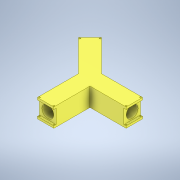
# Autodesk Inventor part: testPrintBracket
Saved by Autodesk Inventor 2022 (Build 260153000, 153)
## iProperties
Created: 2022-02-05
Part Number: testPrintBracket
Material: Generic
Document SubType Name: Modeling
Designer: ultra
Density: 1 g/cm^3
Appearance: Smooth - Yellow
Author: ultra
Autodesk Inventor part; units mm, degrees
ref_plane "YZ Plane" through (0, 0, 0) normal (1, 0, 0) x (0, 1, 0)
ref_plane "XZ Plane" through (0, 0, 0) normal (0, 1, 0) x (-1, 0, 0)
ref_plane "XY Plane" through (0, 0, 0) normal (0, 0, 1) x (1, 0, 0)
sketch "Sketch2" plane through (0, 0, 0) normal (1, 0, 0) x (0, 1, 0)
  circle A0 centre (0, 0) radius 13.2937
  line L0 (-16, -18.5) -> (16, -18.5)
  line L1 (16, -18.5) -> (16, 18.5)
  line L2 (16, 18.5) -> (-16, 18.5)
  line L3 (-16, 18.5) -> (-16, -18.5)
  line L4 (-16, -18.5) -> (16, 18.5) construction
  line L5 (16, -18.5) -> (-16, 18.5) construction
  dimension "d9" = 26.5875
  dimension "d10" = 32
  dimension "d11" = 37
  constraints: 12 end point, 2 midpoint, 2 parallel, 1 centre point, 1 coincident, 1 horizontal, 1 perpendicular
  measures "d9" diameter of A0
  measures "d10" distance of L2.end L1.end
  measures "d11" distance of L1.end L0.end
extrude "Extrusion2" add sketch "Sketch2" along normal blind 76.2
sketch "Sketch3" plane through (0, -16, -18.5) normal (0, 0, -1) x (-1, 0, 0)
  line L0 (0, 0) -> (0, 32) projected
  circle A0 centre (18.5, 16) radius 13.2937
  line L1 (0, 32) -> (0, 0)
  line L2 (0, 0) -> (37, 0)
  line L3 (37, 0) -> (37, 32)
  line L4 (37, 32) -> (0, 32)
  line L5 (0, 32) -> (37, 0) construction
  line L6 (0, 0) -> (37, 32) construction
  point P0 (0, 16)
  dimension "d14" = 26.5875
  dimension "d15" = 32
  dimension "d16" = 37
  constraints: 12 end point, 2 midpoint, 2 parallel, 1 centre point, 1 coincident, 1 perpendicular
  measures "d14" diameter of A0
  measures "d15" distance of L3.end L2.end
  measures "d16" distance of L2.end L1.end
extrude "Extrusion3" add sketch "Sketch3" against normal blind 113.2
sketch "Sketch4" plane through (76.2, -16, -18.5) normal (0, 0, -1) x (-1, 0, 0)
  circle A0 centre (94.7, 16) radius 13.2937 projected
  point P0 (76.2, 16)
extrude "Extrusion4" add sketch "Sketch4" against normal blind 37
sketch "Sketch5" plane through (76.2, 16, 18.5) normal (0, 1, 0) x (1, 0, 0)
  line L0 (-113.2, 37) -> (0, 37) projected
  line L1 (-113.2, 37) -> (-113.2, -76.2) projected
  line L2 (-113.2, 37) -> (-100.1185, 50.0815)
  line L3 (-113.2, 37) -> (-94.7, 37) construction
  line L4 (-113.2, 37) -> (-126.2815, 23.9185)
  line L5 (-113.2, 37) -> (-94.7, 37) construction
  line L6 (-100.1185, 50.0815) -> (-154.0001, 103.963)
  line L7 (-126.2815, 23.9185) -> (-180.163, 77.8001)
  line L8 (-126.2815, 23.9185) -> (-50.0815, 23.9185) construction
  line L9 (-154.0001, 103.963) -> (-180.163, 77.8001)
  line L10 (-100.1185, 50.0815) -> (-87.037, 37)
  line L11 (-126.2815, 23.9185) -> (-113.2, 10.837)
  point P0 (-76.2, 18.5)
  dimension "d21" = 18.5
  dimension "d22" = 45
  dimension "d23" = 18.5
  dimension "d24" = 135
  dimension "d25" = 76.2
  dimension "d26" = 76.2
  dimension "d27" = 135
  constraints: 20 end point, 3 equal length, 3 horizontal, 2 point on line
  measures "d21" distance of L0.start L2.end
  measures "d22" angle of L3 L2
  measures "d23" distance of L0.start L4.end
  measures "d24" angle of L4 L5
  measures "d25" distance of L2.end L6.end
  measures "d26" distance of L4.end L7.end
  measures "d27" angle of L8 L7
extrude "Extrusion5" add sketch "Sketch5" against normal blind 32
sketch "Sketch7" plane through (-77.8001, -16, -85.463) normal (-0.7071068, 0, -0.7071068) x (-0.7071068, 0, 0.7071068)
  line L0 (37, 0) -> (37, 32)
  line L1 (37, 32) -> (0, 32)
  line L2 (0, 32) -> (0, 0)
  line L3 (0, 0) -> (37, 0)
  circle A0 centre (18.5, 16) radius 13.2937
  point P0 (5.4185, 16)
  point P1 (37, 16)
  constraints: 8 end point, 1 centre point
extrude "Extrusion6" cut sketch "Sketch7" against normal blind 101.6 contours A0
sketch "Sketch8" plane through (76.2, 16, 18.5) normal (0, 1, 0) x (1, 0, 0)
  line L0 (-76.2, 0) -> (0, 0) projected
  line L1 (-87.037, 37) -> (0, 37) projected
  line L2 (-87.037, 37) -> (-154.0001, 103.963) projected
  line L3 (-180.163, 77.8001) -> (-113.2, 10.837) projected
  line L4 (-113.2, 10.837) -> (-113.2, -76.2) projected
  line L5 (-76.2, 0) -> (-76.2, -76.2) projected
  line L6 (0, 37) -> (5, 37)
  line L7 (5, 37) -> (5, 0)
  line L8 (5, 0) -> (0, 0)
  line L9 (0, 0) -> (0, 37)
  line L10 (-113.2, -76.2) -> (-76.2, -76.2)
  line L11 (-76.2, -76.2) -> (-76.2, -81.2)
  line L12 (-76.2, -81.2) -> (-113.2, -81.2)
  line L13 (-113.2, -81.2) -> (-113.2, -76.2)
  line L14 (-180.163, 77.8001) -> (-183.6985, 81.3356)
  line L15 (-183.6985, 81.3356) -> (-157.5356, 107.4985)
  line L16 (-157.5356, 107.4985) -> (-154.0001, 103.963)
  point P0 (-76.2, 18.5)
  dimension "d32" = 5
  dimension "d33" = 5
  dimension "d34" = 5
  dimension "d35" = 90
  constraints: 22 end point, 4 parallel, 3 perpendicular, 2 horizontal
  measures "d32" distance of L7.end L8.end
  measures "d33" distance of L10.end L11.end
  measures "d34" distance of L3.start L14.end
  measures "d35" angle of L14 L15
extrude "Extrusion7" add sketch "Sketch8" along normal blind 4.7752
sketch "Sketch9" plane through (76.2, -16, -18.5) normal (0, -1, 0) x (1, 0, 0)
  line L0 (-87.037, 0) -> (0, 0) projected
  line L1 (-76.2, 37) -> (0, 37) projected
  line L2 (-76.2, 37) -> (-76.2, 113.2) projected
  line L3 (-113.2, 26.163) -> (-113.2, 113.2) projected
  line L4 (-113.2, 26.163) -> (-180.163, -40.8001) projected
  line L5 (-154.0001, -66.963) -> (-87.037, 0) projected
  line L6 (-76.2, 118.2) -> (-76.2, 37) projected
  line L7 (-113.2, 113.2) -> (-76.2, 113.2)
  line L8 (-76.2, 113.2) -> (-76.2, 118.2)
  line L9 (-76.2, 118.2) -> (-113.2, 118.2)
  line L10 (-113.2, 118.2) -> (-113.2, 113.2)
  line L11 (-76.2, 37) -> (5, 37) projected
  line L12 (0, 0) -> (5, 0)
  line L13 (5, 0) -> (5, 37)
  line L14 (5, 37) -> (0, 37)
  line L15 (0, 37) -> (0, 0)
  line L16 (-183.6985, -44.3356) -> (-113.2, 26.163) projected
  line L17 (-180.163, -40.8001) -> (-183.6985, -44.3356)
  line L18 (-183.6985, -44.3356) -> (-157.5356, -70.4985)
  line L19 (-157.5356, -70.4985) -> (-154.0001, -66.963)
  point P0 (-76.2, 18.5)
  constraints: 22 end point, 4 parallel, 4 perpendicular, 2 horizontal, 1 collinear
extrude "Extrusion8" add sketch "Sketch9" along normal blind 4.7752
sketch "Sketch10" plane through (76.2, 20.7752, 18.5) normal (0, 1, 0) x (1, 0, 0)
  circle A0 centre (2.5, 34.5) radius 1.5875
  circle A1 centre (2.5, 2.5) radius 1.5875
  line L0 (0, 37) -> (0, 0)
  line L1 (0, 0) -> (5, 0)
  line L2 (5, 37) -> (5, 0)
  line L3 (0, 37) -> (5, 37)
  point P0 (-76.2, 18.5)
  point P1 (0, 18.5)
  constraints: 8 end point, 2 centre point
extrude "Extrusion9" cut sketch "Sketch10" against normal blind 279.4 contours A0 | A1
sketch "Sketch11" plane through (76.2, 20.7752, 18.5) normal (0, 1, 0) x (1, 0, 0)
  circle A0 centre (-78.7, -78.7) radius 1.5875
  circle A1 centre (-110.7, -78.7) radius 1.5875
  line L0 (-76.2, -76.2) -> (-113.2, -76.2)
  line L1 (-113.2, -76.2) -> (-113.2, -81.2)
  line L2 (-76.2, -81.2) -> (-113.2, -81.2)
  line L3 (-76.2, -76.2) -> (-76.2, -81.2)
  circle A2 centre (-157.5356, 103.963) radius 1.5875
  circle A3 centre (-180.163, 81.3356) radius 1.5875
  line L4 (-157.5356, 107.4985) -> (-183.6985, 81.3356)
  line L5 (-183.6985, 81.3356) -> (-180.163, 77.8001)
  line L6 (-154.0001, 103.963) -> (-180.163, 77.8001)
  line L7 (-157.5356, 107.4985) -> (-154.0001, 103.963)
  point P0 (-76.2, 18.5)
  point P1 (-94.7, -76.2)
  point P2 (-170.6171, 94.4171)
  constraints: 16 end point, 4 centre point
extrude "Extrusion10" cut sketch "Sketch11" against normal blind 279.4 contours A0 | A1 | A2 | A3
body "Solid2"
